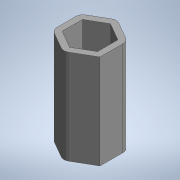
# Autodesk Inventor part: arm wheel spacer
Saved by Autodesk Inventor 2022.3 (Build 263350000, 350)
## iProperties
Part Number: arm wheel spacer
Material: Generic
Document SubType Name: Modeling
Designer: mavericks
Appearance: Default
Author: mavericks
Autodesk Inventor part; units mm, degrees
ref_plane "YZ Plane" through (0, 0, 0) normal (1, 0, 0) x (0, 1, 0)
ref_plane "XZ Plane" through (0, 0, 0) normal (0, 1, 0) x (-1, 0, 0)
ref_plane "XY Plane" through (0, 0, 0) normal (0, 0, 1) x (1, 0, 0)
sketch "Sketch1" plane through (0, 0, 0) normal (0, 1, 0) x (-1, 0, 0)
  line L0 (0, 0) -> (6.35, -3.6662)
  line L1 (6.35, -3.6662) -> (6.35, -10.9985)
  line L2 (6.35, -10.9985) -> (0, -14.6647)
  line L3 (0, -14.6647) -> (-6.35, -10.9985)
  line L4 (-6.35, -10.9985) -> (-6.35, -3.6662)
  line L5 (-6.35, -3.6662) -> (0, 0)
  line L6 (0, 0) -> (0, -14.6647) construction
  line L7 (6.35, -10.9985) -> (-6.35, -3.6662) construction
  line L8 (6.35, -3.6662) -> (-6.35, -10.9985) construction
  line L9 (0, -1.8331) -> (4.7625, -4.5827)
  line L10 (4.7625, -4.5827) -> (4.7625, -10.082)
  line L11 (4.7625, -10.082) -> (0, -12.8316)
  line L12 (0, -12.8316) -> (-4.7625, -10.082)
  line L13 (-4.7625, -10.082) -> (-4.7625, -4.5827)
  line L14 (-4.7625, -4.5827) -> (0, -1.8331)
  line L15 (4.7625, -4.5827) -> (-4.7625, -10.082) construction
  line L16 (0, -12.8316) -> (0, -1.8331) construction
  line L17 (4.7625, -10.082) -> (-4.7625, -4.5827) construction
  point P0 (0, -7.3323)
  dimension "d0" = 12.7
  dimension "d2" = 9.525
  constraints: 36 end point, 12 equal length, 3 vertical, 2 horizontal alignment, 2 midpoint, 2 parallel
  measures "d0" distance between parallel lines of L4 L1
  measures "d2" distance between parallel lines of L13 L10
extrude "Extrusion1" add sketch "Sketch1" along normal blind 25.4
fillet "Fillet1" radius 2 5 edges at (0, 12.7, 0) (-6.35, 12.7, -3.6662) (-6.35, 12.7, -10.9985) (0, 12.7, -14.6647) (6.35, 12.7, -10.9985)
body "Solid1"
